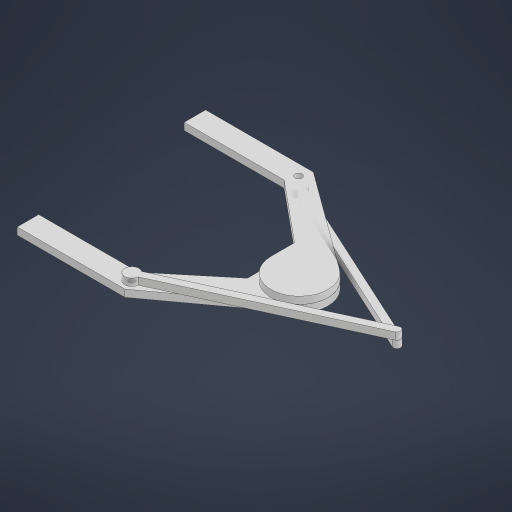
# Autodesk Inventor part: Claw
Saved by Autodesk Inventor 2023 (Build 270158000, 158)
## iProperties
Created: 2023-01-16
Part Number: Claw
Material: Generic
Document SubType Name: Modeling
Designer: Terrence
Density: 1 g/cm^3
Appearance: Default
Author: Terrence
Autodesk Inventor part; units mm, degrees
ref_plane "YZ Plane" through (0, 0, 0) normal (1, 0, 0) x (0, 1, 0)
ref_plane "XZ Plane" through (0, 0, 0) normal (0, 1, 0) x (-1, 0, 0)
ref_plane "XY Plane" through (0, 0, 0) normal (0, 0, 1) x (1, 0, 0)
sketch "Sketch1" plane through (0, 0, 0) normal (0, 1, 0) x (-1, 0, 0)
  circle A0 centre (0, 0) radius 50.8
  circle A1 centre (109, 0) radius 50.8
  line L0 (0, 0) -> (-114.6721, 0) construction
  line L1 (0, 0) -> (156.6813, -129.3879)
  line L2 (415.459, 120.65) -> (174.159, 120.65)
  line L3 (174.159, 120.65) -> (174.159, -120.65)
  line L4 (174.159, -120.65) -> (415.459, -120.65)
  line L5 (415.459, -120.65) -> (415.459, 120.65)
  line L6 (156.6813, -129.3879) -> (334.4813, -129.3879)
  line L7 (334.4813, -167.4879) -> (142.9832, -167.4879)
  line L8 (142.9832, -167.4879) -> (-29.9854, -41.0063)
  line L9 (334.4813, -129.3879) -> (334.4813, -167.4879)
  line L10 (0, 0) -> (156.6813, 129.3879)
  line L11 (156.6813, 129.3879) -> (334.4813, 129.3879)
  line L12 (334.4813, 167.4879) -> (142.9832, 167.4879)
  line L13 (142.9832, 167.4879) -> (-29.9854, 41.0063)
  line L14 (334.4813, 129.3879) -> (334.4813, 167.4879)
  line L15 (0, 0) -> (50.8, 0) construction
  line L16 (50.8, 0) -> (50.8, -41.9508)
  line L17 (50.8, 0) -> (50.8, 41.9508)
  point P0 (174.159, 0)
  point P1 (39.1703, -32.347)
  point P2 (-29.9854, 41.0063)
  point P3 (39.1703, 32.347)
  dimension "d0" = 101.6
  dimension "d1" = 101.6
  dimension "d2" = 203.2
  dimension "d3" = 241.3
  dimension "d4" = 241.3
  dimension "d5" = 177.8
  dimension "d7" = 140.45
  dimension "d8" = 38.1
  dimension "d9" = 38.1
  constraints: 36 end point, 6 symmetric about line, 3 horizontal, 3 point on line, 2 centre point, 2 parallel, 2 point on circle, 2 tangent, 1 coincident, 1 midpoint, 1 perpendicular, 1 vertical
  measures "d0" diameter of A0
  measures "d1" diameter of A1
  measures "d2" distance of L0.start L1.end
  measures "d3" distance of L4.end L3.end
  measures "d4" distance of L3.end L2.end
  measures "d5" distance of L1.end L6.end
  measures "d7" angle of L1 L6
  measures "d8" distance between parallel lines of L6 L7
  measures "d9" distance of L6.end L7.start
extrude "Extrusion1" add sketch "Sketch1" along normal blind 12.7 contours A0 L10 L1 | A0 L1 L6 L9 L7 L8 | A0 L1 L10 | A0 L16 L1
extrude "Extrusion2" add sketch "Sketch1" against normal blind 12.7 separate body contours A0 L10 L1 | L13 L12 L14 L11 L10 A0 | L10 L17 A0 | A0 L1 L10
sketch "Sketch2" plane through (0, 0, 0) normal (0, -1, 0) x (1, 0, 0)
  line L0 (0, 0) -> (374.3117, 0) construction
  line L1 (-156.6813, -129.3879) -> (-142.9832, -167.4879)
  line L2 (-149.8322, -148.4379) -> (173.3048, 0) construction
  line L3 (170.6542, 5.7703) -> (-152.4829, -142.6676)
  line L4 (-152.4829, -142.6676) -> (-147.1816, -154.2082)
  line L5 (-137.1871, -149.6171) -> (175.9555, -5.7703)
  line L6 (175.9555, -5.7703) -> (170.6542, 5.7703)
  line L7 (170.6542, 5.7703) -> (-147.1816, -154.2082) construction
  line L8 (-152.4829, -142.6676) -> (175.9555, -5.7703) construction
  circle A0 centre (-149.8322, -148.4379) radius 12.7
  circle A1 centre (173.3048, 0) radius 6.35
  point P0 (11.7363, -74.2189)
  point P1 (-142.4884, -138.0765)
  point P2 (175.9555, -5.7703)
  dimension "d18" = 25.4
  dimension "d16" = 355.6
  dimension "d17" = 12.7
  dimension "d21" = 12.7
  constraints: 18 end point, 6 midpoint, 3 parallel, 2 coincident, 1 centre point, 1 horizontal, 1 perpendicular, 1 point on line, 3 other
  measures "d16" distance of L2.start L2.end
  measures "d17" distance of L4.end L3.end
  measures "d21" diameter of A1
extrude "Extrusion3" add sketch "Sketch2" along normal blind 12.7 separate body
ref_plane "Work Plane1" through (0, 0, 0) normal (0, 1, 0) x (1, 0, 0)
ref_plane "Work Plane2" through (-334.4813, 0, 0) normal (0, 0, 1) x (1, 0, 0)
mirror "Mirror2" about plane through (0, 0, 0) normal (0, 1, 0) bodies 3 separate body
mirror "Mirror3" about plane through (-334.4813, 0, 0) normal (0, 0, 1) remove original yes bodies 4
sketch "Sketch4" plane through (0, 12.7, 0) normal (0, 1, 0) x (1, 0, 0)
  line L0 (-334.4813, 129.3879) -> (-156.6813, 129.3879) projected
  line L1 (29.9854, 41.0063) -> (-142.9832, 167.4879) projected
  line L2 (-156.6813, 129.3879) -> (-142.9832, 167.4879) construction
  circle A0 centre (-149.8322, 148.4379) radius 6.35
  point P0 (0, 0)
  dimension "d25" = 12.7
  constraints: 2 end point, 1 centre point, 1 coincident, 1 midpoint
  measures "d25" diameter of A0
extrude "Extrusion5" cut sketch "Sketch4" against normal blind 12.7 bodies 1
sketch "Sketch5" plane through (0, -12.7, 0) normal (0, -1, 0) x (1, 0, 0)
  line L0 (-142.9832, 167.4879) -> (-334.4813, 167.4879) projected
  line L1 (-334.4813, 129.3879) -> (-156.6813, 129.3879) projected
  line L2 (-142.9832, 167.4879) -> (-156.6813, 129.3879) construction
  circle A0 centre (-149.8322, 148.4379) radius 6.35
  point P0 (0, 0)
  dimension "d28" = 12.7
  constraints: 2 end point, 1 centre point, 1 coincident, 1 midpoint
  measures "d28" diameter of A0
extrude "Extrusion6" cut sketch "Sketch5" against normal blind 12.7 bodies 2
body "Solid1"
body "Solid2"
body "Solid3"
body "Solid4"
